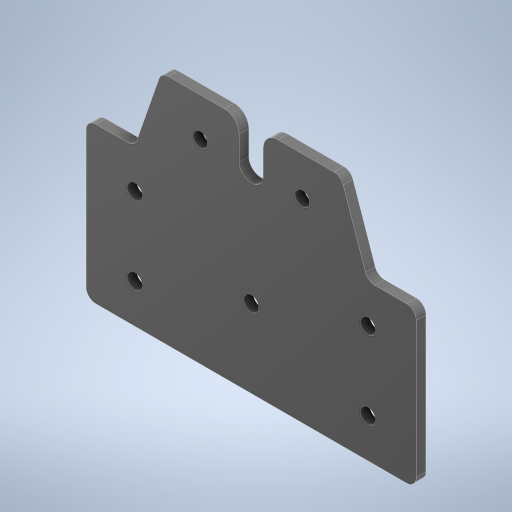
# Autodesk Inventor part: Bumper Plates
Saved by Autodesk Inventor 2023 (Build 270158000, 158)
## iProperties
Created: 2023-11-09
Part Number: Bumper Plates
Material: Generic
Document SubType Name: Modeling
Designer: jackc
Density: 1 g/cm^3
Appearance: Smooth - Black
Author: jackc
Autodesk Inventor part; units mm, degrees
ref_plane "YZ Plane" through (0, 0, 0) normal (1, 0, 0) x (0, 1, 0)
ref_plane "XZ Plane" through (0, 0, 0) normal (0, 1, 0) x (-1, 0, 0)
ref_plane "XY Plane" through (0, 0, 0) normal (0, 0, 1) x (1, 0, 0)
sketch "Sketch1" plane through (0, 0, 0) normal (0, 0, 1) x (1, 0, 0)
  line L0 (0, 0) -> (107.95, 0)
  line L1 (107.95, 0) -> (107.95, 50.8)
  line L2 (107.95, 50.8) -> (92.075, 50.8)
  line L3 (92.075, 50.8) -> (83.3438, 76.2)
  line L4 (83.3438, 76.2) -> (57.9438, 76.2)
  line L5 (57.9438, 76.2) -> (57.9438, 63.5)
  line L6 (50.0063, 63.5) -> (50.0063, 76.2)
  line L7 (50.0063, 76.2) -> (24.6062, 76.2)
  line L8 (24.6062, 76.2) -> (15.875, 50.8)
  line L9 (15.875, 50.8) -> (0, 50.8)
  line L10 (0, 50.8) -> (0, 0)
  circle A0 centre (53.975, 25.4) radius 2.5019
  circle A1 centre (15.875, 38.1) radius 2.5019
  circle A2 centre (15.875, 12.7) radius 2.5019
  circle A3 centre (92.075, 38.1) radius 2.5019
  circle A4 centre (92.075, 12.7) radius 2.5019
  arc A5 (50.0063, 63.5) -> (57.9438, 63.5) centre (53.975, 63.5) ccw
  circle A6 centre (37.3063, 63.5) radius 2.3813
  circle A7 centre (70.6437, 63.5) radius 2.3813
  dimension "d0" = 50.8
  dimension "d1" = 107.95
  dimension "d2" = 7.9375
  dimension "d3" = 53.975
  dimension "d4" = 25.4
  dimension "d5" = 5.0038
  dimension "d6" = 38.1
  dimension "d7" = 12.7
  dimension "d8" = 25.4
  dimension "d9" = 38.1
  dimension "d11" = 25.4
  dimension "d12" = 25.4
  dimension "d14" = 12.7
  dimension "d15" = 4.7625
  dimension "d16" = 4.7625
  dimension "d17" = 12.7
  dimension "d18" = 12.7
  constraints: 22 end point, 8 centre point, 4 equal length, 4 equal radius, 4 horizontal alignment, 3 parallel, 3 perpendicular, 3 vertical alignment, 2 point on circle, 2 point on line, 2 tangent, 1 horizontal, 1 vertical
  measures "d0" distance between parallel lines of L0 L9
  measures "d1" distance of L0.start L0.end
  measures "d2" distance between parallel lines of L5 L6
  measures "d3" distance from line of A0.centre L1
  measures "d4" distance from line of A0.centre L0
  measures "d5" diameter of A0
  measures "d6" horizontal distance of A3.centre A0.centre
  measures "d7" vertical distance of A3.centre A0.centre
  measures "d8" distance of A3.centre A4.centre
  measures "d9" horizontal distance of A0.centre A1.centre
  measures "d11" distance between parallel lines of L4 L2
  measures "d12" distance of L6.end L7.end
  measures "d14" distance from line of A5.centre L4
  measures "d15" diameter of A7
  measures "d16" diameter of A6
  measures "d17" distance from line of L5 A7.centre
  measures "d18" distance from line of A6.centre L6
extrude "Extrusion1" add sketch "Sketch1" along normal blind 3.175
fillet "Fillet1" radius 3.175 8 edges at (15.875, 50.8, 1.5875) (0, 50.8, 1.5875) (0, 0, 1.5875) (107.95, 0, 1.5875) (107.95, 50.8, 1.5875) (92.075, 50.8, 1.5875) (83.3438, 76.2, 1.5875) (24.6062, 76.2, 1.5875)
fillet "Fillet2" radius 4.7625 2 edges at (50.0063, 76.2, 1.5875) (57.9438, 76.2, 1.5875)
equation "\"d16\" = d15"
body "Solid1"
